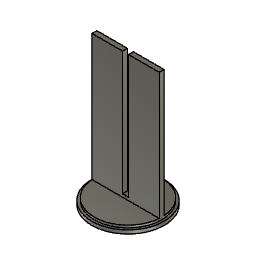
Blank Can with Vertical Shelf V1 (Autodesk Fusion 360 design; units mm, degrees)
Autodesk Fusion 360 part; units mm, degrees
sketch "Base" plane through (0, 0, 0) normal (0, 0, 1) x (1, 0, 0)
  circle A0 centre (0, 0) radius 30
  circle A1 centre (0, 0) radius 28
  dimension "d1" = 60
  dimension "d2" = 56
  constraint coincident A0.centre A1.centre
  constraint concentric A0 A1
  measures "d1" diameter of A0
  measures "d2" diameter of A1
extrude "Extrude1" add sketch "Base" along normal blind 2 contours A1 makes body 1
extrude "Extrude2" add sketch "Base" along normal blind 113 bodies 1
sketch "Sketch2" plane through (0, 0, 0) normal (0, 0, 1) x (1, 0, 0)
  circle A0 centre (0, 0) radius 28
  line L0 (0, -2) -> (27.9285, -2)
  line L1 (-27.9285, -2) -> (0, -2)
  line L2 (0, 2) -> (-27.9285, 2)
  line L3 (27.9285, 2) -> (0, 2)
  circle A1 centre (0, 0) radius 30
  constraint coincident A0.centre A1.centre
  constraint coincident A0 L0.end
  constraint horizontal L0
  constraint coincident A0 L1.start
  constraint parallel L0 L1
  constraint coincident A0 L2.end
  constraint parallel L0 L2
  constraint coincident A0 L3.start
  constraint parallel L2 L3
extrude "Extrude3" add sketch "Sketch2" along normal blind 3 separate body makes body 2
extrude "Extrude4" add sketch "Sketch2" along normal blind 5 contours A0 L0 L1 bodies 2
extrude "Extrude5" add sketch "Sketch2" along normal blind 5 contours A0 L2 L3 bodies 2
extrude "Extrude6" add sketch "Sketch2" along normal blind 110 contours A0 L0 L1 L2 L3 bodies 2
sketch "Sketch6" plane through (0, 2, 0) normal (0, 1, 0) x (-1, 0, 0)
  line L0 (-27.9285, 5) -> (27.9285, 5)
  line L1 (27.9285, 5) -> (27.9285, 110)
  line L2 (27.9285, 110) -> (-27.9285, 110)
  line L3 (-27.9285, 110) -> (-27.9285, 5)
  line L4 (-2.5, 7.5) -> (2.5, 7.5)
  line L5 (2.5, 7.5) -> (2.5, 110)
  line L6 (-2.5, 110) -> (2.5, 110)
  line L7 (-2.5, 110) -> (-2.5, 7.5)
  dimension "d15" = 102.5
  dimension "d16" = 5
  constraint parallel L0 L4
  constraint coincident L2 L5.end
  constraint perpendicular L2 L5
  constraint coincident L2 L6.start
  constraint perpendicular L4 L7
  measures "d15" distance of L4.end L5.end
  measures "d16" distance of L5.end L6.start
extrude "Extrude7" cut sketch "Sketch6" against normal blind 4 contours L2 L4 L5 L6 L7 bodies 2
hidden bodies 1
named bodies: "Bottom"
